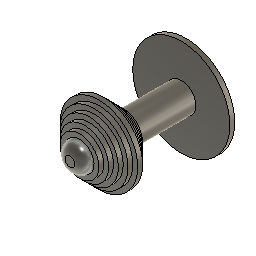
Doorknobs_final_subtract (Autodesk Fusion 360 design; units mm, degrees)
Autodesk Fusion 360 part; units mm, degrees
sketch "Sketch1" plane through (0, 0, 0) normal (1, 0, 0) x (0, 1, 0) in component "Doorknob_Revolve_Addition"
  line L0 (0, 0) -> (0, 31.75)
  line L1 (-25.4, 3.175) -> (-25.4, 6.35)
  line L2 (-31.75, 6.35) -> (-31.75, 12.7)
  line L3 (-31.75, 12.7) -> (-38.1, 12.7)
  line L4 (-38.1, 12.7) -> (-38.1, 19.05)
  line L5 (-25.4, 6.35) -> (-31.75, 6.35)
  line L6 (-38.1, 19.05) -> (-44.45, 19.05)
  line L7 (-44.45, 19.05) -> (-44.45, 25.4)
  line L8 (-44.45, 25.4) -> (-50.8, 25.4)
  line L9 (-50.8, 25.4) -> (-50.8, 19.05)
  line L10 (-50.8, 19.05) -> (-57.15, 19.05)
  line L11 (-57.15, 19.05) -> (-57.15, 12.7)
  line L12 (-57.15, 12.7) -> (-63.5, 12.7)
  line L13 (-63.5, 12.7) -> (-63.5, 6.35)
  line L14 (-63.5, 6.35) -> (-69.85, 6.35)
  line L15 (-69.85, 6.35) -> (-69.85, 4.7625)
  line L16 (-76.2, 0) -> (0, 0)
  arc A0 (-69.85, 4.7625) -> (-76.2, 0) centre (-69.85, -1.8521) ccw
  line L17 (-69.85, 4.7625) -> (-69.85, -1.8521) construction
  line L18 (-69.85, 4.7625) -> (-25.4, 4.7625) construction
  line L19 (0, 31.75) -> (-3.175, 31.75)
  line L20 (-3.175, 31.75) -> (-3.175, 3.175)
  line L21 (-3.175, 3.175) -> (-25.4, 3.175)
  dimension "d4" = 76.2
  dimension "d5" = 31.75
  dimension "d6" = 25.4
  dimension "d10" = 6.35
  dimension "d11" = 6.35
  dimension "d12" = 6.35
  dimension "d13" = 6.35
  dimension "d14" = 6.35
  dimension "d15" = 6.35
  dimension "d16" = 6.35
  dimension "d23" = 3.175
  dimension "d24" = 22.225
  dimension "d25" = 3.175
  constraint coincident L0.start L16.end
  constraint vertical L0
  constraint parallel L0 L2
  constraint perpendicular L0 L3
  constraint perpendicular L3 L4
  constraint perpendicular L1 L5
  constraint perpendicular L4 L6
  constraint perpendicular L6 L7
  constraint perpendicular L7 L8
  constraint perpendicular L8 L9
  constraint perpendicular L9 L10
  constraint perpendicular L10 L11
  constraint perpendicular L9 L12
  constraint perpendicular L12 L13
  constraint perpendicular L9 L14
  constraint perpendicular L14 L15
  constraint horizontal L16
  constraint collinear L5 L14
  constraint collinear L3 L12
  constraint collinear L6 L10
  constraint equal L5 L14
  constraint equal L3 L12
  constraint equal L6 L10
  constraint coincident A0.centre L17.end
  constraint vertical L17
  constraint midpoint L1 L18.end
  constraint horizontal L18
  constraint perpendicular L0 L19
  constraint horizontal L21
  constraint vertical L20
  measures "d4" distance of L0.start L16.start
  measures "d5" distance of L0.start L0.end
  measures "d6" distance of L8 L16
  measures "d10" distance of L6 L8
  measures "d11" distance of L3.end L4.end
  measures "d12" distance of L2.start L2.end
  measures "d13" distance of L7.end L8.end
  measures "d14" distance of L4.end L6.end
  measures "d15" distance of L2.end L3.end
  measures "d16" distance of L1.end L2.start
  measures "d23" distance of L0.end L19.end
  measures "d24" distance of L1.start L20.end
  measures "d25" distance of L16 L21
revolve "Revolve1" add sketch "Sketch1" angle 360 about axis through (0, -76.2, 0) along (0, 1, 0) makes body 1 in component "Doorknob_Revolve_Addition"
cylinder "CylinderPrimitive1" add diameter 63.5 height 76.2 placed x (1, 0, 0) y (0, 0, -1) z (0, 1, 0) at (0, 0, 0) separate body makes body 2 in component "Doorknob_Revolve_Subtract"
sketch "Sketch4" plane through (0, 0, 0) normal (1, 0, 0) x (0, 1, 0) in component "Doorknob_Revolve_Subtract"
  line L0 (76.2, -31.75) -> (76.2, 31.75)
  line L1 (73.025, 31.75) -> (73.025, 9.525)
  line L2 (73.025, 9.525) -> (34.925, 9.525)
  line L3 (34.925, 9.525) -> (34.925, 12.7)
  line L4 (34.925, 12.7) -> (31.75, 12.7)
  line L5 (31.75, 12.7) -> (31.75, 15.875)
  line L6 (31.75, 15.875) -> (28.575, 15.875)
  line L7 (28.575, 15.875) -> (28.575, 19.05)
  line L8 (28.575, 19.05) -> (25.4, 19.05)
  line L9 (25.4, 19.05) -> (25.4, 22.225)
  line L10 (25.4, 22.225) -> (22.225, 22.225)
  line L11 (22.225, 22.225) -> (22.225, 25.4)
  line L12 (22.225, 25.4) -> (19.05, 25.4)
  line L13 (19.05, 25.4) -> (19.05, 22.225)
  line L14 (19.05, 22.225) -> (15.875, 22.225)
  line L15 (15.875, 22.225) -> (15.875, 19.05)
  line L16 (15.875, 19.05) -> (12.7, 19.05)
  line L17 (12.7, 19.05) -> (12.7, 15.875)
  line L18 (12.7, 15.875) -> (9.525, 15.875)
  line L19 (9.525, 15.875) -> (9.525, 12.7)
  line L20 (0, 31.75) -> (0, -31.75)
  line L21 (9.525, 12.7) -> (6.35, 12.7)
  line L22 (6.35, 12.7) -> (6.35, 9.525)
  line L23 (6.35, 9.525) -> (0, 9.525)
  line L24 (0, -31.75) -> (76.2, -31.75)
  line L25 (76.2, 31.75) -> (0, 31.75)
  dimension "d29" = 9.525
  dimension "d30" = 3.175
  dimension "d31" = 3.175
  dimension "d32" = 3.175
  dimension "d33" = 3.175
  dimension "d34" = 3.175
  dimension "d35" = 3.175
  dimension "d36" = 38.1
  dimension "d37" = 3.175
  dimension "d38" = 3.175
  dimension "d39" = 3.175
  dimension "d40" = 3.175
  dimension "d41" = 3.175
  dimension "d42" = 25.4
  constraint parallel L0 L1
  constraint perpendicular L1 L2
  constraint perpendicular L2 L3
  constraint perpendicular L3 L4
  constraint perpendicular L4 L5
  constraint perpendicular L5 L6
  constraint perpendicular L6 L7
  constraint perpendicular L7 L8
  constraint perpendicular L8 L9
  constraint perpendicular L9 L10
  constraint perpendicular L10 L11
  constraint perpendicular L9 L12
  constraint perpendicular L10 L13
  constraint perpendicular L13 L14
  constraint perpendicular L14 L15
  constraint perpendicular L13 L16
  constraint perpendicular L16 L17
  constraint perpendicular L17 L18
  constraint perpendicular L18 L19
  constraint perpendicular L19 L21
  constraint collinear L10 L14
  constraint collinear L8 L16
  constraint collinear L6 L18
  constraint collinear L4 L21
  constraint perpendicular L21 L22
  constraint perpendicular L20 L23
  constraint collinear L2 L23
  constraint equal L10 L14
  constraint equal L8 L16
  constraint equal L6 L18
  constraint equal L4 L21
  constraint coincident L20 L23.end
  constraint coincident L25 L1.start
  measures "d29" distance of origin L23
  measures "d30" distance of L21.end L22.end
  measures "d31" distance of L18.end L19.end
  measures "d32" distance of L16.end L17.end
  measures "d33" distance of L14.end L15.end
  measures "d34" distance of L12.end L13.end
  measures "d35" distance of L0 L1
  measures "d36" distance of L1.end L2.end
  measures "d37" distance of L3.end L4.end
  measures "d38" distance of L5.end L6.end
  measures "d39" distance of L7.end L8.end
  measures "d40" distance of L9.end L10.end
  measures "d41" distance of L11.end L12.end
  measures "d42" distance of origin L12
revolve "Revolve1'" cut sketch "Sketch4" angle 360 about axis through (0, 1.75, 0) along (0, 1, 0) contours L1 L2 L3 L4 L5 L6 L7 L8 L9 L10 L11 L12 L13 L14 L15 L16 L17 L18 L19 L20 L21 L22 L23 L25 bodies 2 in component "Doorknob_Revolve_Subtract"
fillet "Fillet1" radius 6.35 1 edges at (3.4444, 0, -8.8804) on bodies 2 in component "Doorknob_Revolve_Subtract"
component "Doorknob_Revolve_Addition" placed x (1, 0, 0) y (0, 1, 0) z (0, 0, 1) at (0, 0, 0)
component "Doorknob_Revolve_Subtract" placed x (1, 0, 0) y (0, 1, 0) z (0, 0, 1) at (0, 0, 0)
equation "d5 = ( 2.5 / 2 ) * 1 in"
equation "d11 = d10"
equation "d12 = d10"
equation "d14 = d13"
equation "d15 = d14"
equation "d16 = d13"
equation "d31 = d30"
equation "d32 = d30"
equation "d33 = d30"
equation "d34 = d30"
equation "d38 = d37"
equation "d39 = d37"
equation "d40 = d37"
equation "d41 = d37"
